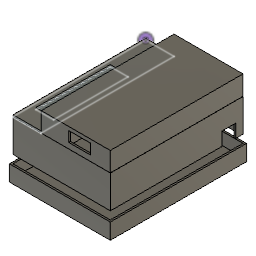
New Pico DMX Panel (Autodesk Fusion 360 design; units mm, degrees)
part number: 2025-12-26-20-46-20-408
Autodesk Fusion 360 part; units mm, degrees
sketch "Button Panel" plane through (0, 0, 0) normal (0, 0, 1) x (1, 0, 0)
  line L0 (0, 0) -> (16, 0)
  line L1 (16, 0) -> (16, -75)
  line L2 (16, -75) -> (0, -75)
  line L3 (0, -75) -> (0, 0)
  line L4 (3, -65) -> (13, -65)
  line L5 (13, -65) -> (13, -23)
  line L6 (13, -23) -> (3, -23)
  line L7 (3, -23) -> (3, -65)
  dimension "d1" = 75
  dimension "d2" = 16
  dimension "d41" = 10
  dimension "d42" = 42
  dimension "d43" = 3
  dimension "d44" = 10
  constraint horizontal L0
  constraint vertical L1
  constraint horizontal L2
  constraint vertical L3
  constraint coincident L0.start L3.end
  constraint horizontal L4
  constraint vertical L5
  constraint horizontal L6
  constraint vertical L7
  measures "d1" distance of L0 L2
  measures "d2" distance of L1 L3
  measures "d41" distance of L4.start L4.end
  measures "d42" distance of L4.start L6.end
  measures "d43" distance of L3 L7
  measures "d44" distance of L2 L4
extrude "Extrude2" add sketch "Button Panel" along normal blind 1 makes body 1
sketch "Pico Housing" plane through (0, 0, 0) normal (0, 0, 1) x (1, 0, 0)
  line L0 (16, 0) -> (55, 0)
  line L1 (55, 0) -> (55, -75)
  line L2 (55, -75) -> (16, -75)
  line L3 (16, -75) -> (16, 0)
  dimension "d20" = 39
  dimension "d39" = 75
  constraint horizontal L0
  constraint vertical L1
  constraint horizontal L2
  constraint vertical L3
  measures "d20" distance of L0.start L0.end
  measures "d39" distance of L0 L2
extrude "Extrude3" add sketch "Pico Housing" along normal blind 9 thin wall 1 inside bodies 1
sketch "Sketch4" plane through (0, 0, 9) normal (0, 0, 1) x (-1, 0, 0)
  line L0 (-17, 74) -> (-17, 1)
  line L1 (-17, 1) -> (-54, 1)
  line L2 (-54, 1) -> (-54, 74)
  line L3 (-54, 74) -> (-17, 74)
  line L4 (-16, 75) -> (-55, 75)
  line L5 (-55, 75) -> (-55, 0)
  line L6 (-55, 0) -> (-16, 0)
  line L7 (-16, 0) -> (-16, 75)
  line L8 (-16, 0) -> (-55, 0)
  line L9 (-55, 0) -> (-55, 75)
  line L10 (-55, 75) -> (-16, 75)
  line L11 (-16, 75) -> (-16, 0)
  constraint horizontal L8
  constraint vertical L9
  constraint horizontal L10
  constraint vertical L11
  constraint coincident L4.end L5.start
  constraint coincident L6.end L7.start
extrude "Extrude4" add sketch "Sketch4" along normal blind 2 contours L0 L1 L2 L3 | L4 L5 L6 L7 L8 L9 L10 L11 bodies 1
sketch "Sketch5" plane through (0, -75, 0) normal (0, -1, 0) x (1, 0, 0)
  line L0 (0, 0) -> (55, 0)
  line L1 (55, 0) -> (55, 11)
  line L2 (55, 11) -> (16, 11)
  line L3 (16, 11) -> (16, 1)
  line L4 (31.5, 10.7) -> (43.8, 10.7)
  line L5 (43.8, 10.7) -> (43.8, 3.2)
  line L6 (43.8, 3.2) -> (31.5, 3.2)
  line L7 (31.5, 3.2) -> (31.5, 10.7)
  line L8 (16, 1) -> (0, 1)
  line L9 (0, 1) -> (0, 0)
  dimension "d26" = 12.3
  dimension "d27" = 7.5
  dimension "d28" = 11.2
  dimension "d29" = 0.3
  constraint horizontal L4
  constraint vertical L5
  constraint horizontal L6
  constraint vertical L7
  measures "d26" distance of L4.start L4.end
  measures "d27" distance of L4.start L6.end
  measures "d28" distance of L1 L5
  measures "d29" distance of L2 L4
extrude "Extrude5" cut sketch "Sketch5" against normal blind 2 contours L4 L5 L6 L7 bodies 1
extrude "Extrude6" add 1 faces at (35.6, -73, 10.1333) along direction (0, -1, 0) blind 2 on bodies 1 bodies 1
sketch "Sketch6" plane through (0, 0, 0) normal (0, 0, 1) x (1, 0, 0)
  line L0 (0, -74.9802) -> (55.0615, -74.9802)
  line L1 (55.0615, -74.9802) -> (55.0615, 0.0198)
  line L2 (55.0615, 0.0198) -> (0, 0.0198)
  line L3 (0, 0.0198) -> (0, -74.9802)
  dimension "d40" = 75
  constraint horizontal L0
  constraint vertical L1
  constraint horizontal L2
  constraint vertical L3
  measures "d40" distance of L0 L2
extrude "Extrude7" add sketch "Sketch6" against normal blind 18.5 thin wall 1 inside bodies 1
sketch "Sketch7" plane through (55.0615, 0, 0) normal (1, 0, 0) x (0, 1, 0)
  line L0 (0.0198, -18.5) -> (0.0198, 0)
  line L1 (-74.9802, 0) -> (-74.9802, -18.5)
  line L2 (-4.246, -18.5) -> (-12, -18.5)
  line L3 (-12, -18.5) -> (-12, -11)
  line L4 (-12, -11) -> (-4.246, -11)
  line L5 (-4.246, -11) -> (-4.246, -18.5)
  line L6 (0.0198, 0) -> (-74.9802, 0)
  line L7 (-74.9802, -18.5) -> (0.0198, -18.5)
  constraint horizontal L2
  constraint vertical L3
  constraint horizontal L4
  constraint vertical L5
extrude "Extrude8" cut sketch "Sketch7" against normal blind 2 contours L2 L3 L4 L5 L7 bodies 1
extrude "Extrude9" add sketch "Button Panel" against normal blind 2 separate body contours L4 L5 L6 L7 makes body 2
extrude "Extrude10" add sketch "Button Panel" against normal blind 2 separate body contours L4 L5 L6 L7 makes body 3
box "BoxPrimitive1" add length 77 width 57 height 2 placed x (0, -1, 0) y (1, 0, 0) z (0, 0, 1) at (-2, 0, 0) separate body makes body 4
move_body "Move1" bodies 4 to x (1, 0, 0) y (0, 1, 0) z (0, 0, 1) at (0, 0, -25)
move_face "MoveFace1" by (0, 0, -7) 1 faces at (17, -77, -24.3333) on bodies 4
move_body "Move2" bodies 4 to x (1, 0, 0) y (0, 1, 0) z (0, 0, 1) at (0, 0, -7)
extrude "Extrude11" add 1 faces at (36, -25.6667, -30) along direction (0, 0, 1) blind 7 thin wall 1 inside on bodies 4 bodies 4
move_body "Move3" bodies 4 to x (1, 0, 0) y (0, 1, 0) z (0, 0, 1) at (2, 2, 0)
move_body "Move4" bodies 4 to x (1, 0, 0) y (0, 1, 0) z (0, 0, 1) at (-1, -3, 0)
move_body "Move5" bodies 4 to x (1, 0, 0) y (0, 1, 0) z (0, 0, 1) at (0, 1, 0)
move_body "Move6" bodies 4 to x (1, 0, 0) y (0, 1, 0) z (0, 0, 1) at (0, 1, 0)
named bodies: "Bottom Panel"
